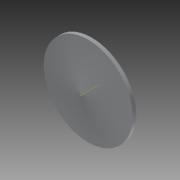
# Autodesk Inventor part: Magnifying Glass
Saved by Autodesk Inventor 2014 (Build 180170000, 170)
## iProperties
Created: 2014-08-03
Part Number: Magnifying Glass
Material: Glass
Document SubType Name: Modeling
Designer: steele
Density: 2.18 g/cm^3
Appearance: Clear
Author: steele
Autodesk Inventor part; units mm, degrees
ref_plane "YZ Plane" through (0, 0, 0) normal (1, 0, 0) x (0, 1, 0)
ref_plane "XZ Plane" through (0, 0, 0) normal (0, 1, 0) x (-1, 0, 0)
ref_plane "XY Plane" through (0, 0, 0) normal (0, 0, 1) x (1, 0, 0)
sketch "Sketch1" plane through (0, 0, 0) normal (0, 0, 1) x (1, 0, 0)
  line L0 (0, 0) -> (0, 9)
  line L1 (0, 0) -> (50, 0) construction
  line L2 (50, 0) -> (50, 2)
  line L3 (0, 9) -> (50, 2)
  line L4 (0, 0) -> (0, -9)
  line L5 (50, 0) -> (50, -2)
  line L6 (0, -9) -> (50, -2)
  line L7 (0, -12.6) -> (0, 12.6) projected
  dimension "d0" = 50
  dimension "d1" = 9
  dimension "d2" = 2
  constraints: 14 end point, 2 perpendicular, 2 symmetric about line
  measures "d0" distance of L0.start L1.end
  measures "d1" distance of L0.start L0.end
  measures "d2" distance of L1.end L2.end
revolve "Revolution1" add sketch "Sketch1" angle 360 about axis through (0, -10, 0) along (0, 1, 0)
body "Solid1"
